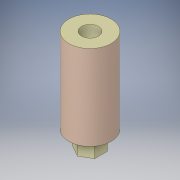
# Autodesk Inventor part: separator
Saved by Autodesk Inventor 2019 (Build 230136000, 136)
## iProperties
Created: 2019-04-09
Part Number: separator
Material: PET Plastic
Document SubType Name: Modeling
Designer: jmc
Density: 1.541 g/cm^3
Appearance: Smooth - Ash
Author: jmc
Autodesk Inventor part; units mm, degrees
ref_plane "YZ Plane" through (0, 0, 0) normal (1, 0, 0) x (0, 1, 0)
ref_plane "XZ Plane" through (0, 0, 0) normal (0, 1, 0) x (-1, 0, 0)
ref_plane "XY Plane" through (0, 0, 0) normal (0, 0, 1) x (1, 0, 0)
sketch "Sketch1" plane through (0, 0, 0) normal (0, 1, 0) x (-1, 0, 0)
  circle A0 centre (0, 0) radius 1.5 construction
  line L0 (0, -1.5) -> (-1.299, -0.75)
  line L1 (-1.299, -0.75) -> (-1.299, 0.75)
  line L2 (-1.299, 0.75) -> (0, 1.5)
  line L3 (0, 1.5) -> (1.299, 0.75)
  line L4 (1.299, 0.75) -> (1.299, -0.75)
  line L5 (1.299, -0.75) -> (0, -1.5)
  dimension "d0" = 3
  constraints: 12 end point, 2 coincident, 1 vertical alignment, 15 other
extrude "Extrusion1" add sketch "Sketch1" along normal blind 2
sketch "Sketch2" plane through (0, 2, 0) normal (0, 1, 0) x (1, 0, 0)
  circle A0 centre (0, 0) radius 2.5
  dimension "d3" = 5
  constraints: 1 centre point, 1 coincident
  measures "d3" diameter of A0
extrude "Extrusion2" add sketch "Sketch2" along normal blind 10
sketch "Sketch3" plane through (0, 12, 0) normal (0, 1, 0) x (1, 0, 0)
  circle A0 centre (0, 0) radius 2.5 projected
  constraints: 1 coincident
hole "Hole1" at (0, 12, 0) direction (0, -1, 0) diameter 2 end through all
body "Solid1"
